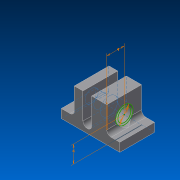
# Autodesk Inventor part: ethernet card support
Saved by Autodesk Inventor 2015 (Build 190159000, 159)
## iProperties
Created: 2017-03-23
Part Number: ethernet card support
Material: Generic
Document SubType Name: Modeling
Designer: ZigZagJoe
Density: 1 g/cm^3
Appearance: Default
Author: ZigZagJoe
Autodesk Inventor part; units mm, degrees
ref_plane "YZ Plane" through (0, 0, 0) normal (1, 0, 0) x (0, 1, 0)
ref_plane "XZ Plane" through (0, 0, 0) normal (0, 1, 0) x (-1, 0, 0)
ref_plane "XY Plane" through (0, 0, 0) normal (0, 0, 1) x (1, 0, 0)
sketch "Sketch1" plane through (0, 0, 0) normal (0, 1, 0) x (-1, 0, 0)
  line L0 (1.9826, -0.2694) -> (1.9826, -7.2694)
  line L1 (1.9826, -7.2694) -> (-0.0174, -7.2694)
  line L2 (-0.0174, -7.2694) -> (-0.0174, -0.2694)
  line L3 (-0.0174, -0.2694) -> (-3.5174, -0.2694)
  line L4 (-3.5174, -0.2694) -> (-3.5174, -8.2694)
  line L5 (-3.5174, -8.2694) -> (3.9826, -8.2694)
  line L6 (3.9826, -8.2694) -> (3.9826, -0.2694)
  line L7 (3.9826, -0.2694) -> (1.9826, -0.2694)
  line L8 (-3.5174, -8.2694) -> (-7.5174, -8.2694)
  line L9 (-7.5174, -8.2694) -> (-7.5174, -4.2694)
  line L10 (-7.5174, -4.2694) -> (-3.5174, -4.2694)
  line L11 (-3.5174, -4.2694) -> (-3.5174, -8.2694)
  line L12 (3.9826, -8.2694) -> (6.9826, -8.2694)
  line L13 (6.9826, -8.2694) -> (6.9826, -6.2694)
  line L14 (6.9826, -6.2694) -> (3.9826, -6.2694)
  line L15 (3.9826, -6.2694) -> (3.9826, -8.2694)
  line L16 (-3.5174, -8.2694) -> (-6.5174, -8.2694)
  line L17 (-6.5174, -8.2694) -> (-6.5174, -6.2694)
  line L18 (-6.5174, -6.2694) -> (-3.5174, -6.2694)
  line L19 (-3.5174, -6.2694) -> (-3.5174, -8.2694)
  point P0 (0, 0)
  dimension "d0" = 2
  dimension "d1" = 3.5
  dimension "d2" = 2
  dimension "d5" = 1
  dimension "d6" = 7
  dimension "d7" = 4
  dimension "d8" = 4
  dimension "d18" = 3
  dimension "d19" = 3
  dimension "d24" = 2
  constraints: 40 end point, 10 perpendicular, 6 parallel, 3 horizontal, 2 point on line, 1 vertical
  measures "d0" distance of L0.end L1.end
  measures "d1" distance of L2.end L3.end
  measures "d2" distance of L6.end L0.start
  measures "d5" distance between parallel lines of L5 L1
  measures "d6" distance of L1.end L2.end
  measures "d7" distance of L9.end L10.end
  measures "d8" distance of L8.end L9.end
  measures "d18" distance of L14.end L13.end
  measures "d19" distance of L17.end L18.end
  measures "d24" distance of L12.end L13.end
extrude "Extrusion1" add sketch "Sketch1" along normal blind 8 contours L7 L6 L5 L4 L3 L2 L1 L0 | L14 L13 L12 L6 | L8 L17 L18 L4
sketch "Sketch2" plane through (7.5174, 0, -8.2694) normal (0, 0, -1) x (-1, 0, 0)
  circle A0 centre (4, 4) radius 2.05
  line L0 (0, 0) -> (0, 8) projected
  line L1 (1, 8) -> (14.5, 8) projected
  line L2 (7.5, 0) -> (7.5, 8) projected
  point P0 (7.5174, 0)
  point P1 (12, 8)
  dimension "d11" = 4.1
  dimension "d12" = 4
  dimension "d13" = 4
  dimension "d17" = 3.5
  constraints: 1 centre point
  measures "d11" diameter of A0
  measures "d12" distance from line of L0 A0.centre
  measures "d13" distance from line of L1 A0.centre
  measures "d17" distance from line of L2 A0.centre
extrude "Extrusion2" [suppressed]
fillet "Fillet1" radius 1 4 edges at (-1.9826, 4, -7.2694) (0.0174, 4, -7.2694) (3.5174, 4, -6.2694) (-3.9826, 4, -6.2694)
sketch "Sketch3" plane through (3.5174, 0, -0.2694) normal (1, 0, 0) x (0, 0, -1)
  circle A0 centre (4, 4) radius 2
  circle A1 centre (4, 4) radius 1.5
  line L0 (8, 0) -> (8, 8) projected
  line L1 (0, 0) -> (5, 0) projected
  point P0 (-0.2694, 0)
  dimension "d20" = 4
  dimension "d21" = 3
  dimension "d22" = 4
  dimension "d23" = 4
  constraints: 2 centre point, 1 coincident
  measures "d20" diameter of A0
  measures "d21" diameter of A1
  measures "d22" distance from line of L0 A0.centre
  measures "d23" distance from line of L1 A0.centre
extrude "Extrusion3" cut sketch "Sketch3" against normal blind 10 contours A1
extrude "Extrusion4" cut sketch "Sketch3" against normal blind 3.5
extrude "Extrusion5" cut sketch "Sketch3" along normal blind 3.5 contours A0 | A1
body "Solid1"
